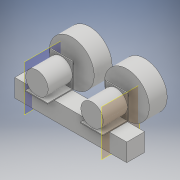
# Autodesk Inventor part: BSF_Accelerator_v01
Saved by Autodesk Inventor 2018 (Build 220112000, 112)
## iProperties
Created: 2019-03-24
Part Number: BSF_Accelerator_v01
Material: Generic
Document SubType Name: Modeling
Designer: simon
Density: 1 g/cm^3
Appearance: Default
Author: simon
Autodesk Inventor part; units mm, degrees
ref_plane "YZ Plane" through (0, 0, 0) normal (1, 0, 0) x (0, 1, 0)
ref_plane "XZ Plane" through (0, 0, 0) normal (0, 1, 0) x (-1, 0, 0)
ref_plane "XY Plane" through (0, 0, 0) normal (0, 0, 1) x (1, 0, 0)
sketch "Sketch1" plane through (0, 0, 0) normal (0, 0, 1) x (1, 0, 0)
  line L0 (-125, 20) -> (125, 20)
  line L1 (125, 20) -> (125, -20)
  line L2 (125, -20) -> (-125, -20)
  line L3 (-125, -20) -> (-125, 20)
  line L4 (-125, 20) -> (125, -20) construction
  line L5 (125, 20) -> (-125, -20) construction
  point P0 (0, 0)
  dimension "d0" = 250
  dimension "d1" = 40
  constraints: 12 end point, 2 midpoint, 2 parallel, 1 horizontal, 1 perpendicular
  measures "d0" distance of L1.end L2.end
  measures "d1" distance of L0.end L1.end
extrude "Extrusion1" add sketch "Sketch1" along normal blind 40
sketch "Sketch2" plane through (-125, 20, 0) normal (0, 1, 0) x (1, 0, 0)
  circle A0 centre (63.5, -68) radius 25
  circle A1 centre (186.5, -68) radius 25
  line L0 (250, -40) -> (0, -40) projected
  line L1 (0, 0) -> (0, -40) projected
  line L2 (250, 0) -> (250, -40) projected
  point P0 (125, 0)
  dimension "d4" = 50
  dimension "d5" = 50
  dimension "d6" = 28
  dimension "d7" = 28
  dimension "d8" = 63.5
  dimension "d9" = 63.5
  dimension "d10" = 123
  constraints: 2 centre point
  measures "d4" diameter of A0
  measures "d5" diameter of A1
  measures "d6" distance from line of L0 A0.centre
  measures "d7" distance from line of L0 A1.centre
  measures "d8" distance from line of A0.centre L1
  measures "d9" distance from line of L2 A1.centre
  measures "d10" distance of A1.centre A0.centre
extrude "Extrusion2" add sketch "Sketch2" against normal blind 54
sketch "Sketch3" plane through (-61.5, 20, 68) normal (0, 1, 0) x (1, 0, 0)
  circle A0 centre (0, 0) radius 4
  circle A1 centre (123, 0) radius 25 projected
  circle A2 centre (123, 0) radius 4
  point P0 (61.5, 68)
  dimension "d13" = 8
  dimension "d14" = 8
  constraints: 2 centre point, 1 coincident
  measures "d13" diameter of A0
  measures "d14" diameter of A2
extrude "Extrusion3" add sketch "Sketch3" along normal blind 23.8 contours A0 | A2
ref_plane "Work Plane1" through (-86.5, 20, 68) normal (-1, 0, 0) x (0, -1, 0)
ref_plane "Work Plane2" through (86.5, 20, 68) normal (1, 0, 0) x (0, 1, 0)
sketch "Sketch5" plane through (-86.5, 20, 68) normal (-1, 0, 0) x (0, -1, 0)
  line L0 (0, -28) -> (55, -28)
  line L1 (55, -28) -> (55, -26)
  line L2 (55, -26) -> (0, -26)
  line L3 (0, -26) -> (0, -28)
  line L4 (0, -28) -> (-2, -28)
  line L5 (-2, -28) -> (-2, 27)
  line L6 (-2, 27) -> (0, 27)
  line L7 (0, 27) -> (0, -28)
  point P0 (20, -68)
  dimension "d17" = 55
  dimension "d18" = 2
  dimension "d19" = 2
  dimension "d20" = 55
  constraints: 16 end point, 4 parallel, 2 horizontal, 2 perpendicular
  measures "d17" distance of L2.end L1.end
  measures "d18" distance of L1.end L0.end
  measures "d19" distance of L5.end L6.end
  measures "d20" distance of L4.end L5.end
extrude "Extrusion4" add sketch "Sketch5" against normal blind 50
sketch "Sketch6" plane through (86.5, 20, 68) normal (1, 0, 0) x (0, 1, 0)
  line L0 (0, 27) -> (0, 0) projected
  line L1 (0, 0) -> (0, -26) projected
  line L2 (0, -26) -> (-55, -26) projected
  line L3 (-55, -26) -> (-55, -28) projected
  line L4 (-55, -28) -> (-40, -28) projected
  line L5 (0, -28) -> (-40, -28) projected
  line L6 (0, -28) -> (2, -28) projected
  line L7 (2, -28) -> (2, 27) projected
  line L8 (2, 27) -> (0, 27) projected
  point P0 (-20, -68)
extrude "Extrusion5" add sketch "Sketch6" against normal blind 50
sketch "Sketch7" plane through (-61.5, 43.8, 68) normal (0, 1, 0) x (1, 0, 0)
  circle A0 centre (0, 0) radius 4 projected
  circle A1 centre (0, 0) radius 50
  circle A2 centre (123, 0) radius 4 projected
  circle A3 centre (123, 0) radius 50
  point P0 (61.5, 68)
  dimension "d25" = 100
  dimension "d26" = 100
  constraints: 2 centre point, 2 coincident
  measures "d25" diameter of A1
  measures "d26" diameter of A3
extrude "Extrusion6" add sketch "Sketch7" along normal blind 40
equation "\"d7\" = d6"
equation "\"d9\" = d8"
body "Solid1"
